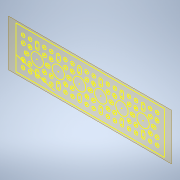
# Autodesk Inventor part: shooter side
Saved by Autodesk Inventor 2021 (Build 250183000, 183)
## iProperties
Created: 2021-04-03
Part Number: shooter side
Material: Generic
Document SubType Name: Modeling
Designer: deli
Density: 1 g/cm^3
Appearance: Default
Author: deli
Autodesk Inventor part; units mm, degrees
ref_plane "YZ Plane" through (0, 0, 0) normal (1, 0, 0) x (0, 1, 0)
ref_plane "XZ Plane" through (0, 0, 0) normal (0, 1, 0) x (-1, 0, 0)
ref_plane "XY Plane" through (0, 0, 0) normal (0, 0, 1) x (1, 0, 0)
ref_plane "Work Plane1" through (0, 0, 0) normal (0, 0, 1) x (1, 0, 0)
sketch "Sketch1" plane through (0, 0, 0) normal (0, 0, 1) x (1, 0, 0)
  line L0 (168, 0) -> (168, 48) projected
  line L1 (0, 48) -> (168, 48) projected
  line L2 (0, 0) -> (0, 48) projected
  line L3 (0, 0) -> (168, 0) projected
  circle A0 centre (144, 24) radius 7 projected
  circle A1 centre (120, 24) radius 7 projected
  arc A2 (136.9289, 33.8995) -> (134.1005, 31.0711) centre (135.5147, 32.4853) ccw projected
  line L4 (137.4142, 33.4142) -> (136.9289, 33.8995) projected
  arc A3 (134.5858, 30.5858) -> (137.4142, 33.4142) centre (136, 32) ccw projected
  line L5 (134.1005, 31.0711) -> (134.5858, 30.5858) projected
  line L6 (132.6863, 26) -> (131.3137, 26) projected
  arc A4 (132.6863, 22) -> (132.6863, 26) centre (132.6863, 24) ccw projected
  line L7 (131.3137, 22) -> (132.6863, 22) projected
  arc A5 (131.3137, 26) -> (131.3137, 22) centre (131.3137, 24) ccw projected
  arc A6 (134.1005, 16.9289) -> (136.9289, 14.1005) centre (135.5147, 15.5147) ccw projected
  line L8 (134.5858, 17.4142) -> (134.1005, 16.9289) projected
  arc A7 (137.4142, 14.5858) -> (134.5858, 17.4142) centre (136, 16) ccw projected
  line L9 (136.9289, 14.1005) -> (137.4142, 14.5858) projected
  arc A8 (153.8995, 31.0711) -> (151.0711, 33.8995) centre (152.4853, 32.4853) ccw projected
  line L10 (153.4142, 30.5858) -> (153.8995, 31.0711) projected
  arc A9 (150.5858, 33.4142) -> (153.4142, 30.5858) centre (152, 32) ccw projected
  line L11 (151.0711, 33.8995) -> (150.5858, 33.4142) projected
  arc A10 (156.6863, 22) -> (156.6863, 26) centre (156.6863, 24) ccw projected
  line L12 (155.3137, 22) -> (156.6863, 22) projected
  arc A11 (155.3137, 26) -> (155.3137, 22) centre (155.3137, 24) ccw projected
  line L13 (156.6863, 26) -> (155.3137, 26) projected
  line L14 (146, 35.3137) -> (146, 40) projected
  arc A12 (142, 35.3137) -> (146, 35.3137) centre (144, 35.3137) ccw projected
  line L15 (142, 40) -> (142, 35.3137) projected
  arc A13 (146, 40) -> (142, 40) centre (144, 40) ccw projected
  circle A14 centre (136, 40) radius 2 projected
  circle A15 centre (128, 40) radius 2 projected
  line L16 (122, 35.3137) -> (122, 40) projected
  arc A16 (118, 35.3137) -> (122, 35.3137) centre (120, 35.3137) ccw projected
  line L17 (118, 40) -> (118, 35.3137) projected
  arc A17 (122, 40) -> (118, 40) centre (120, 40) ccw projected
  circle A18 centre (112, 40) radius 2 projected
  circle A19 centre (104, 40) radius 2 projected
  line L18 (98, 35.3137) -> (98, 40) projected
  arc A20 (94, 35.3137) -> (98, 35.3137) centre (96, 35.3137) ccw projected
  line L19 (94, 40) -> (94, 35.3137) projected
  arc A21 (98, 40) -> (94, 40) centre (96, 40) ccw projected
  circle A22 centre (88, 40) radius 2 projected
  circle A23 centre (80, 40) radius 2 projected
  line L20 (74, 35.3137) -> (74, 40) projected
  arc A24 (70, 35.3137) -> (74, 35.3137) centre (72, 35.3137) ccw projected
  line L21 (70, 40) -> (70, 35.3137) projected
  arc A25 (74, 40) -> (70, 40) centre (72, 40) ccw projected
  circle A26 centre (64, 40) radius 2 projected
  circle A27 centre (56, 40) radius 2 projected
  line L22 (50, 35.3137) -> (50, 40) projected
  arc A28 (46, 35.3137) -> (50, 35.3137) centre (48, 35.3137) ccw projected
  line L23 (46, 40) -> (46, 35.3137) projected
  arc A29 (50, 40) -> (46, 40) centre (48, 40) ccw projected
  circle A30 centre (40, 40) radius 2 projected
  circle A31 centre (32, 40) radius 2 projected
  line L24 (26, 35.3137) -> (26, 40) projected
  arc A32 (22, 35.3137) -> (26, 35.3137) centre (24, 35.3137) ccw projected
  line L25 (22, 40) -> (22, 35.3137) projected
  arc A33 (26, 40) -> (22, 40) centre (24, 40) ccw projected
  circle A34 centre (16, 40) radius 2 projected
  circle A35 centre (8, 40) radius 2 projected
  line L26 (142, 12.6863) -> (142, 8) projected
  arc A36 (146, 12.6863) -> (142, 12.6863) centre (144, 12.6863) ccw projected
  line L27 (146, 8) -> (146, 12.6863) projected
  arc A37 (142, 8) -> (146, 8) centre (144, 8) ccw projected
  circle A38 centre (136, 8) radius 2 projected
  circle A39 centre (128, 8) radius 2 projected
  line L28 (118, 12.6863) -> (118, 8) projected
  arc A40 (122, 12.6863) -> (118, 12.6863) centre (120, 12.6863) ccw projected
  line L29 (122, 8) -> (122, 12.6863) projected
  arc A41 (118, 8) -> (122, 8) centre (120, 8) ccw projected
  circle A42 centre (112, 8) radius 2 projected
  circle A43 centre (104, 8) radius 2 projected
  line L30 (94, 12.6863) -> (94, 8) projected
  arc A44 (98, 12.6863) -> (94, 12.6863) centre (96, 12.6863) ccw projected
  line L31 (98, 8) -> (98, 12.6863) projected
  arc A45 (94, 8) -> (98, 8) centre (96, 8) ccw projected
  circle A46 centre (88, 8) radius 2 projected
  circle A47 centre (80, 8) radius 2 projected
  line L32 (70, 12.6863) -> (70, 8) projected
  arc A48 (74, 12.6863) -> (70, 12.6863) centre (72, 12.6863) ccw projected
  line L33 (74, 8) -> (74, 12.6863) projected
  arc A49 (70, 8) -> (74, 8) centre (72, 8) ccw projected
  circle A50 centre (64, 8) radius 2 projected
  circle A51 centre (56, 8) radius 2 projected
  line L34 (46, 12.6863) -> (46, 8) projected
  arc A52 (50, 12.6863) -> (46, 12.6863) centre (48, 12.6863) ccw projected
  line L35 (50, 8) -> (50, 12.6863) projected
  arc A53 (46, 8) -> (50, 8) centre (48, 8) ccw projected
  circle A54 centre (40, 8) radius 2 projected
  circle A55 centre (32, 8) radius 2 projected
  line L36 (22, 12.6863) -> (22, 8) projected
  arc A56 (26, 12.6863) -> (22, 12.6863) centre (24, 12.6863) ccw projected
  line L37 (26, 8) -> (26, 12.6863) projected
  arc A57 (22, 8) -> (26, 8) centre (24, 8) ccw projected
  circle A58 centre (16, 8) radius 2 projected
  circle A59 centre (8, 8) radius 2 projected
  arc A60 (9.8995, 31.0711) -> (7.0711, 33.8995) centre (8.4853, 32.4853) ccw projected
  line L38 (9.4142, 30.5858) -> (9.8995, 31.0711) projected
  arc A61 (6.5858, 33.4142) -> (9.4142, 30.5858) centre (8, 32) ccw projected
  line L39 (7.0711, 33.8995) -> (6.5858, 33.4142) projected
  arc A62 (7.0711, 14.1005) -> (9.8995, 16.9289) centre (8.4853, 15.5147) ccw projected
  line L40 (6.5858, 14.5858) -> (7.0711, 14.1005) projected
  arc A63 (9.4142, 17.4142) -> (6.5858, 14.5858) centre (8, 16) ccw projected
  line L41 (9.8995, 16.9289) -> (9.4142, 17.4142) projected
  arc A64 (160.9289, 33.8995) -> (158.1005, 31.0711) centre (159.5147, 32.4853) ccw projected
  line L42 (161.4142, 33.4142) -> (160.9289, 33.8995) projected
  arc A65 (158.5858, 30.5858) -> (161.4142, 33.4142) centre (160, 32) ccw projected
  line L43 (158.1005, 31.0711) -> (158.5858, 30.5858) projected
  arc A66 (158.1005, 16.9289) -> (160.9289, 14.1005) centre (159.5147, 15.5147) ccw projected
  line L44 (158.5858, 17.4142) -> (158.1005, 16.9289) projected
  arc A67 (161.4142, 14.5858) -> (158.5858, 17.4142) centre (160, 16) ccw projected
  line L45 (160.9289, 14.1005) -> (161.4142, 14.5858) projected
  circle A68 centre (152, 8) radius 2 projected
  circle A69 centre (152, 40) radius 2 projected
  circle A70 centre (160, 40) radius 2 projected
  circle A71 centre (160, 8) radius 2 projected
  arc A72 (33.8995, 31.0711) -> (31.0711, 33.8995) centre (32.4853, 32.4853) ccw projected
  line L46 (33.4142, 30.5858) -> (33.8995, 31.0711) projected
  arc A73 (30.5858, 33.4142) -> (33.4142, 30.5858) centre (32, 32) ccw projected
  line L47 (31.0711, 33.8995) -> (30.5858, 33.4142) projected
  arc A74 (57.8995, 31.0711) -> (55.0711, 33.8995) centre (56.4853, 32.4853) ccw projected
  line L48 (57.4142, 30.5858) -> (57.8995, 31.0711) projected
  arc A75 (54.5858, 33.4142) -> (57.4142, 30.5858) centre (56, 32) ccw projected
  line L49 (55.0711, 33.8995) -> (54.5858, 33.4142) projected
  arc A76 (81.8995, 31.0711) -> (79.0711, 33.8995) centre (80.4853, 32.4853) ccw projected
  line L50 (81.4142, 30.5858) -> (81.8995, 31.0711) projected
  arc A77 (78.5858, 33.4142) -> (81.4142, 30.5858) centre (80, 32) ccw projected
  line L51 (79.0711, 33.8995) -> (78.5858, 33.4142) projected
  arc A78 (105.8995, 31.0711) -> (103.0711, 33.8995) centre (104.4853, 32.4853) ccw projected
  line L52 (105.4142, 30.5858) -> (105.8995, 31.0711) projected
  arc A79 (102.5858, 33.4142) -> (105.4142, 30.5858) centre (104, 32) ccw projected
  line L53 (103.0711, 33.8995) -> (102.5858, 33.4142) projected
  arc A80 (129.8995, 31.0711) -> (127.0711, 33.8995) centre (128.4853, 32.4853) ccw projected
  line L54 (129.4142, 30.5858) -> (129.8995, 31.0711) projected
  arc A81 (126.5858, 33.4142) -> (129.4142, 30.5858) centre (128, 32) ccw projected
  line L55 (127.0711, 33.8995) -> (126.5858, 33.4142) projected
  arc A82 (14.1005, 16.9289) -> (16.9289, 14.1005) centre (15.5147, 15.5147) ccw projected
  line L56 (14.5858, 17.4142) -> (14.1005, 16.9289) projected
  arc A83 (17.4142, 14.5858) -> (14.5858, 17.4142) centre (16, 16) ccw projected
  line L57 (16.9289, 14.1005) -> (17.4142, 14.5858) projected
  arc A84 (38.1005, 16.9289) -> (40.9289, 14.1005) centre (39.5147, 15.5147) ccw projected
  line L58 (38.5858, 17.4142) -> (38.1005, 16.9289) projected
  arc A85 (41.4142, 14.5858) -> (38.5858, 17.4142) centre (40, 16) ccw projected
  line L59 (40.9289, 14.1005) -> (41.4142, 14.5858) projected
  arc A86 (62.1005, 16.9289) -> (64.9289, 14.1005) centre (63.5147, 15.5147) ccw projected
  line L60 (62.5858, 17.4142) -> (62.1005, 16.9289) projected
  arc A87 (65.4142, 14.5858) -> (62.5858, 17.4142) centre (64, 16) ccw projected
  line L61 (64.9289, 14.1005) -> (65.4142, 14.5858) projected
  arc A88 (86.1005, 16.9289) -> (88.9289, 14.1005) centre (87.5147, 15.5147) ccw projected
  line L62 (86.5858, 17.4142) -> (86.1005, 16.9289) projected
  arc A89 (89.4142, 14.5858) -> (86.5858, 17.4142) centre (88, 16) ccw projected
  line L63 (88.9289, 14.1005) -> (89.4142, 14.5858) projected
  arc A90 (110.1005, 16.9289) -> (112.9289, 14.1005) centre (111.5147, 15.5147) ccw projected
  line L64 (110.5858, 17.4142) -> (110.1005, 16.9289) projected
  arc A91 (113.4142, 14.5858) -> (110.5858, 17.4142) centre (112, 16) ccw projected
  line L65 (112.9289, 14.1005) -> (113.4142, 14.5858) projected
  line L66 (11.3137, 22) -> (12.6863, 22) projected
  arc A92 (11.3137, 26) -> (11.3137, 22) centre (11.3137, 24) ccw projected
  line L67 (12.6863, 26) -> (11.3137, 26) projected
  arc A93 (12.6863, 22) -> (12.6863, 26) centre (12.6863, 24) ccw projected
  line L68 (36.6863, 26) -> (35.3137, 26) projected
  arc A94 (36.6863, 22) -> (36.6863, 26) centre (36.6863, 24) ccw projected
  line L69 (35.3137, 22) -> (36.6863, 22) projected
  arc A95 (35.3137, 26) -> (35.3137, 22) centre (35.3137, 24) ccw projected
  line L70 (60.6863, 26) -> (59.3137, 26) projected
  arc A96 (60.6863, 22) -> (60.6863, 26) centre (60.6863, 24) ccw projected
  line L71 (59.3137, 22) -> (60.6863, 22) projected
  arc A97 (59.3137, 26) -> (59.3137, 22) centre (59.3137, 24) ccw projected
  line L72 (84.6863, 26) -> (83.3137, 26) projected
  arc A98 (84.6863, 22) -> (84.6863, 26) centre (84.6863, 24) ccw projected
  line L73 (83.3137, 22) -> (84.6863, 22) projected
  arc A99 (83.3137, 26) -> (83.3137, 22) centre (83.3137, 24) ccw projected
  line L74 (108.6863, 26) -> (107.3137, 26) projected
  arc A100 (108.6863, 22) -> (108.6863, 26) centre (108.6863, 24) ccw projected
  line L75 (107.3137, 22) -> (108.6863, 22) projected
  arc A101 (107.3137, 26) -> (107.3137, 22) centre (107.3137, 24) ccw projected
  arc A102 (16.9289, 33.8995) -> (14.1005, 31.0711) centre (15.5147, 32.4853) ccw projected
  line L76 (17.4142, 33.4142) -> (16.9289, 33.8995) projected
  arc A103 (14.5858, 30.5858) -> (17.4142, 33.4142) centre (16, 32) ccw projected
  line L77 (14.1005, 31.0711) -> (14.5858, 30.5858) projected
  arc A104 (40.9289, 33.8995) -> (38.1005, 31.0711) centre (39.5147, 32.4853) ccw projected
  line L78 (41.4142, 33.4142) -> (40.9289, 33.8995) projected
  arc A105 (38.5858, 30.5858) -> (41.4142, 33.4142) centre (40, 32) ccw projected
  line L79 (38.1005, 31.0711) -> (38.5858, 30.5858) projected
  arc A106 (64.9289, 33.8995) -> (62.1005, 31.0711) centre (63.5147, 32.4853) ccw projected
  line L80 (65.4142, 33.4142) -> (64.9289, 33.8995) projected
  arc A107 (62.5858, 30.5858) -> (65.4142, 33.4142) centre (64, 32) ccw projected
  line L81 (62.1005, 31.0711) -> (62.5858, 30.5858) projected
  arc A108 (88.9289, 33.8995) -> (86.1005, 31.0711) centre (87.5147, 32.4853) ccw projected
  line L82 (89.4142, 33.4142) -> (88.9289, 33.8995) projected
  arc A109 (86.5858, 30.5858) -> (89.4142, 33.4142) centre (88, 32) ccw projected
  line L83 (86.1005, 31.0711) -> (86.5858, 30.5858) projected
  arc A110 (112.9289, 33.8995) -> (110.1005, 31.0711) centre (111.5147, 32.4853) ccw projected
  line L84 (113.4142, 33.4142) -> (112.9289, 33.8995) projected
  arc A111 (110.5858, 30.5858) -> (113.4142, 33.4142) centre (112, 32) ccw projected
  line L85 (110.1005, 31.0711) -> (110.5858, 30.5858) projected
  arc A112 (31.0711, 14.1005) -> (33.8995, 16.9289) centre (32.4853, 15.5147) ccw projected
  line L86 (30.5858, 14.5858) -> (31.0711, 14.1005) projected
  arc A113 (33.4142, 17.4142) -> (30.5858, 14.5858) centre (32, 16) ccw projected
  line L87 (33.8995, 16.9289) -> (33.4142, 17.4142) projected
  arc A114 (55.0711, 14.1005) -> (57.8995, 16.9289) centre (56.4853, 15.5147) ccw projected
  line L88 (54.5858, 14.5858) -> (55.0711, 14.1005) projected
  arc A115 (57.4142, 17.4142) -> (54.5858, 14.5858) centre (56, 16) ccw projected
  line L89 (57.8995, 16.9289) -> (57.4142, 17.4142) projected
  arc A116 (79.0711, 14.1005) -> (81.8995, 16.9289) centre (80.4853, 15.5147) ccw projected
  line L90 (78.5858, 14.5858) -> (79.0711, 14.1005) projected
  arc A117 (81.4142, 17.4142) -> (78.5858, 14.5858) centre (80, 16) ccw projected
  line L91 (81.8995, 16.9289) -> (81.4142, 17.4142) projected
  arc A118 (103.0711, 14.1005) -> (105.8995, 16.9289) centre (104.4853, 15.5147) ccw projected
  line L92 (102.5858, 14.5858) -> (103.0711, 14.1005) projected
  arc A119 (105.4142, 17.4142) -> (102.5858, 14.5858) centre (104, 16) ccw projected
  line L93 (105.8995, 16.9289) -> (105.4142, 17.4142) projected
  arc A120 (127.0711, 14.1005) -> (129.8995, 16.9289) centre (128.4853, 15.5147) ccw projected
  line L94 (126.5858, 14.5858) -> (127.0711, 14.1005) projected
  arc A121 (129.4142, 17.4142) -> (126.5858, 14.5858) centre (128, 16) ccw projected
  line L95 (129.8995, 16.9289) -> (129.4142, 17.4142) projected
  arc A122 (151.0711, 14.1005) -> (153.8995, 16.9289) centre (152.4853, 15.5147) ccw projected
  line L96 (150.5858, 14.5858) -> (151.0711, 14.1005) projected
  arc A123 (153.4142, 17.4142) -> (150.5858, 14.5858) centre (152, 16) ccw projected
  line L97 (153.8995, 16.9289) -> (153.4142, 17.4142) projected
  circle A124 centre (24, 24) radius 7 projected
  circle A125 centre (48, 24) radius 7 projected
  circle A126 centre (72, 24) radius 7 projected
  circle A127 centre (96, 24) radius 7 projected
  line L98 (168, 24) -> (-50.2098, 24)
  line L99 (-21.6738, 25.907) -> (54.2558, 1.907)
  line L100 (166, 46) -> (2, 46)
  line L101 (2, 46) -> (2, 2)
  line L102 (2, 2) -> (168, 2)
  line L103 (54.409, 14.409) -> (54.8943, 13.9237)
  arc A128 (54.8943, 13.9237) -> (58.0763, 17.1057) centre (56.4853, 15.5147) ccw
  line L104 (58.0763, 17.1057) -> (57.591, 17.591)
  arc A129 (57.591, 17.591) -> (54.409, 14.409) centre (56, 16) ccw
  arc A130 (157.9237, 17.1057) -> (161.1057, 13.9237) centre (159.5147, 15.5147) ccw
  line L105 (157.9237, 17.1057) -> (158.409, 17.591)
  arc A131 (161.591, 14.409) -> (158.409, 17.591) centre (160, 16) ccw
  line L106 (161.591, 14.409) -> (161.1057, 13.9237)
  point P0 (-15.6405, 24)
  point P1 (53.9616, 2)
  dimension "d1" = 2
  dimension "d2" = 0.25
  dimension "d3" = 0.25
  constraints: 18 end point, 8 point on circle, 4 centre point, 1 horizontal, 1 midpoint, 1 point on line, 7 other
  measures "d1" distance between parallel lines of L3 L102
  measures "d2" radial gap between concentric circles of A115 A129
  measures "d3" radial gap between concentric circles of A66 A130
extrude "Extrusion1" add sketch "Sketch1" along normal blind 12.7 contours L102 L99 A54 A55 L37 A56 L36 A82 L57 A83 L56 A62 L41 A63 L101 L98 A92 L66 A93 A124 A95 L69 A94 A125 A97 L71 A96 A126 A99 L73 A98 A127 A101 L75 A100 A1 A5 L7 A4 A0 A11 L12 A10 L0 | L99 L98 L2 | L2 L98 L101 L99 | A10 L12 A11 L98 | L99 A54 | A63 L41 A62 L99 | A0 L98 | L99 A55 | L98 A93 L66 A92 | A82 L56 A83 L57 L99 | A4 L7 A5 L98 | L99 L36 A56 L37 | L98 A124 | A1 L98 | L98 A94 L69 A95 | A100 L75 A101 L98 | L98 A125 | A127 L98 | L98 A96 L71 A97 | A98 L73 A99 L98 | L98 A126 | L8 A7 L9 A6 | A36 L27 A37 L26 | A38 | A39 | A40 L29 A41 L28 | A42 | A43 | A44 L31 A45 L30 | A46 | A47 | A48 L33 A49 L32 | A50 | A51 | A52 L35 A53 L34 | A68 | A71 | L58 A85 L59 A84 | L60 A87 L61 A86 | L62 A89 L63 A88 | L64 A91 L65 A90 | L86 A113 L87 A112 | L90 A117 L91 A116 | L92 A119 L93 A118 | L94 A121 L95 A120 | L96 A123 L97 A122 picked at (40.4231, 8.1099) picked at (145.645, 19.4481) picked at (32.4577, 9.177) picked at (22.475, 20.4369) picked at (119.7187, 21.6837) picked at (47.7187, 21.6837) picked at (95.7187, 21.6837) picked at (71.7187, 21.6837)
sketch "Sketch2" plane through (-15.6405, 24, 0) normal (0, 1, 0) x (1, 0, 0)
  line L0 (183.6405, 0) -> (0, 0) projected
  line L1 (0, 0) -> (50, -12.7)
  line L2 (183.6405, 0) -> (0, 0) projected
  line L3 (0, 0) -> (0, -12.7) projected
  line L4 (183.6405, -12.7) -> (0, -12.7) projected
  line L5 (183.6405, 0) -> (183.6405, -12.7) projected
  line L6 (183.6405, -12.7) -> (0, -12.7) projected
  point P0 (15.6405, 0)
  point P1 (0, 0)
  dimension "d6" = 50
  constraints: 2 end point, 1 point on line
  measures "d6" horizontal distance of L1.end L0.end
extrude "Extrusion2" cut sketch "Sketch2" against normal blind 25 contours L1 L4 L3
fillet "Fillet1" radius 20 1 edges at (34.3595, 16.0979, 12.7)
sketch "Sketch4" plane through (0, 0, 12.7) normal (0, 0, 1) x (1, 0, 0)
  line L0 (36.8598, 7.4056) -> (36.8598, 24) projected
  line L1 (36.8598, 7.4056) -> (53.9616, 2) projected
  line L2 (53.9616, 2) -> (168, 2) projected
  line L3 (168, 2) -> (168, 24) projected
  line L4 (168, 24) -> (36.8598, 24) projected
  line L5 (161.591, 14.409) -> (161.1057, 13.9237) projected
  arc A0 (157.9237, 17.1057) -> (161.1057, 13.9237) centre (159.5147, 15.5147) ccw projected
  line L6 (157.9237, 17.1057) -> (158.409, 17.591) projected
  arc A1 (161.591, 14.409) -> (158.409, 17.591) centre (160, 16) ccw projected
  arc A2 (57.591, 17.591) -> (54.409, 14.409) centre (56, 16) ccw projected
  line L7 (57.591, 17.591) -> (58.0763, 17.1057) projected
  arc A3 (54.8943, 13.9237) -> (58.0763, 17.1057) centre (56.4853, 15.5147) ccw projected
  line L8 (54.8943, 13.9237) -> (54.409, 14.409) projected
  line L9 (59.4905, 18.5199) -> (59.0052, 19.0052)
  arc A4 (59.0052, 19.0052) -> (52.9948, 12.9948) centre (56, 16) ccw
  line L10 (52.9948, 12.9948) -> (53.4801, 12.5095)
  arc A5 (53.4801, 12.5095) -> (59.4905, 18.5199) centre (56.4853, 15.5147) ccw
  line L11 (156.9948, 19.0052) -> (156.5095, 18.5199)
  arc A6 (156.5095, 18.5199) -> (162.5199, 12.5095) centre (159.5147, 15.5147) ccw
  line L12 (162.5199, 12.5095) -> (163.0052, 12.9948)
  arc A7 (163.0052, 12.9948) -> (156.9948, 19.0052) centre (160, 16) ccw
  point P0 (0, 0)
  dimension "d10" = 2
  dimension "d11" = 2
  constraints: 8 end point, 8 point on circle, 4 centre point, 6 other
  measures "d10" radial gap between concentric circles of A3 A5
  measures "d11" radial gap between concentric circles of A1 A7
extrude "Extrusion3" cut sketch "Sketch4" against normal blind 8.7 contours A5 L10 A4 L9 | A7 L12 A6 L11
body "Solid1"
